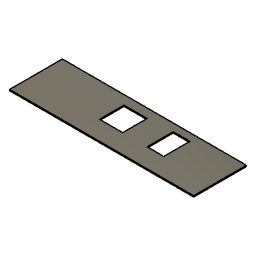
Bauwagen Seite lang (andere Seite) Deichsel rechts v1 (Autodesk Fusion 360 design; units mm, degrees)
Autodesk Fusion 360 part; units mm, degrees
sketch "Skizze1" plane through (0, 0, 0) normal (0, 1, 0) x (1, 0, 0)
  line L0 (0, 0) -> (827, 0)
  line L1 (827, 0) -> (827, -237)
  line L2 (827, -237) -> (0, -237)
  line L3 (0, -237) -> (0, 0)
  line L4 (0, -237) -> (0, -151)
  line L5 (0, -151) -> (318, -151)
  line L6 (318, -151) -> (422, -151)
  line L7 (422, -151) -> (422, -41)
  line L8 (422, -41) -> (318, -41)
  line L9 (318, -41) -> (318, -151)
  line L10 (422, -151) -> (532, -151)
  line L11 (532, -151) -> (607, -151)
  line L12 (607, -151) -> (607, -34)
  line L13 (607, -34) -> (532, -34)
  line L14 (532, -34) -> (532, -151)
  dimension "d1" = 827
  dimension "d2" = 237
  dimension "d3" = 86
  dimension "d4" = 318
  dimension "d5" = 104
  dimension "d6" = 110
  dimension "d7" = 110
  dimension "d8" = 75
  dimension "d9" = 117
  constraint horizontal L0
  constraint vertical L1
  constraint horizontal L2
  constraint vertical L3
  constraint coincident L0.start L3.end
  constraint perpendicular L2 L4
  constraint perpendicular L3 L5
  constraint horizontal L6
  constraint vertical L7
  constraint horizontal L8
  constraint vertical L9
  constraint perpendicular L7 L10
  constraint horizontal L11
  constraint vertical L12
  constraint horizontal L13
  constraint vertical L14
  measures "d1" distance of L0.start L0.end
  measures "d2" distance of L0.start L2.end
  measures "d3" distance of L2.end L4.end
  measures "d4" distance of L4.end L5.end
  measures "d5" distance of L5.end L6.end
  measures "d6" distance of L5.end L8.end
  measures "d7" distance of L6.end L10.end
  measures "d8" distance of L10.end L11.end
  measures "d9" distance of L10.end L13.end
extrude "Extrusion1" add sketch "Skizze1" along normal blind 5
